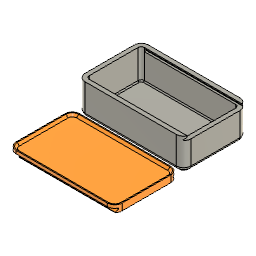
Box+with+Slide+Lid (Autodesk Fusion 360 design; units mm, degrees)
part number: 2025-07-16-15-57-53-406
Autodesk Fusion 360 part; units mm, degrees
note: some values were not read from the file. Set by a fixed rule: which face or edge a step refers to.
sketch "Sketch1" plane through (0, 0, 0) normal (0, 0, 1) x (1, 0, 0)
  line L0 (7, 0) -> (93, 0)
  line L1 (100, 7) -> (100, 53)
  line L2 (93, 60) -> (7, 60)
  line L3 (0, 53) -> (0, 7)
  arc A0 (7, 60) -> (0, 53) centre (7, 53) ccw
  arc A1 (100, 53) -> (93, 60) centre (93, 53) ccw
  arc A2 (93, 0) -> (100, 7) centre (93, 7) ccw
  arc A3 (0, 7) -> (7, 0) centre (7, 7) ccw
  point P0 (100, 0)
  point P1 (0, 60)
  dimension "d5" = 60
  dimension "d6" = 100
  dimension "d7" = 7
  constraint horizontal L0
  constraint vertical L1
  constraint horizontal L2
  constraint vertical L3
  constraint coincident P1 L2
  constraint coincident P1 L3
  constraint tangent L2 A0
  constraint tangent L3 A0
  constraint tangent L1 A1
  constraint tangent L2 A1
  constraint coincident P0 L0
  constraint coincident P0 L1
  constraint tangent L0 A2
  constraint tangent L1 A2
  constraint equal A1 A2
  constraint coincident origin L0
  constraint coincident origin L3
  constraint tangent L0 A3
  constraint tangent L3 A3
  constraint equal A1 A3
  constraint equal A0 A1
  measures "d5" distance of origin P1
  measures "d6" distance of origin P0
  measures "d7" radius of A0
extrude "Extrude1" add sketch "Sketch1" along normal blind 30 makes body 1
shell "Shell1" thickness 4 removed faces 1 at (64.3333, 20, 30) on bodies 1
extrude "Extrude2" cut 1 faces at (64.3333, 21.3333, 4) along direction (0, 0, -1) blind 2 on bodies 1 bodies 1
chamfer "Chamfer1" distance 3 angle 45 8 edges at (2.0503, 2.0503, 0) (50, 0, 0) (97.9497, 2.0503, 0) (100, 30, 0) (97.9497, 57.9497, 0) (50, 60, 0) (2.0503, 57.9497, 0) (0, 30, 0) on bodies 1
fillet "Fillet1" radius 3 8 edges at (2.0503, 57.9497, 3) (50, 60, 3) (97.9497, 57.9497, 3) (100, 30, 3) (97.9497, 2.0503, 3) (50, 0, 3) (2.0503, 2.0503, 3) (0, 30, 3) on bodies 1
chamfer "Chamfer2" distance 1 distance2 1 8 edges at (50, 56, 2) (95.1213, 55.1213, 2) (96, 30, 2) (95.1213, 4.8787, 2) (50, 4, 2) (4.8787, 4.8787, 2) (4, 30, 2) (4.8787, 55.1213, 2) measured on face at (35.6667, 56, 20.6667) measured on face at (94.3747, 55.6665, 11.3333) measured on face at (96, 22.3333, 11.3333) measured on face at (93.2852, 4.0136, 20.6667) measured on face at (35.6667, 4, 11.3333) measured on face at (4.0034, 6.8573, 20.6667) measured on face at (4, 22.3333, 20.6667) measured on face at (5.5, 55.5981, 20.6667) on bodies 1
sketch "Sketch5" plane through (0, 0, 0) normal (0, 0, 1) x (1, 0, 0)
  line L0 (7, -5) -> (93, -5)
  line L1 (100, -12) -> (100, -58)
  line L2 (93, -65) -> (7, -65)
  line L3 (0, -58) -> (0, -12)
  arc A0 (7, -5) -> (0, -12) centre (7, -12) ccw
  arc A1 (100, -12) -> (93, -5) centre (93, -12) ccw
  arc A2 (93, -65) -> (100, -58) centre (93, -58) ccw
  arc A3 (0, -58) -> (7, -65) centre (7, -58) ccw
  point P0 (0, -5)
  point P1 (100, -5)
  point P2 (0, -65)
  dimension "d37" = 100
  dimension "d38" = 60
  dimension "d39" = 5
  dimension "d40" = 7
  constraint horizontal L0
  constraint vertical L1
  constraint horizontal L2
  constraint vertical L3
  constraint coincident P0 L0
  constraint coincident P0 L3
  constraint tangent L0 A0
  constraint tangent L3 A0
  constraint coincident P1 L0
  constraint coincident P1 L1
  constraint tangent L0 A1
  constraint tangent L1 A1
  constraint tangent L1 A2
  constraint tangent L2 A2
  constraint equal A0 A2
  constraint coincident P2 L2
  constraint coincident P2 L3
  constraint tangent L2 A3
  constraint tangent L3 A3
  constraint equal A0 A1
  constraint equal A0 A3
  constraint vertical P0 origin
  measures "d37" distance of P0 P1
  measures "d38" distance of P0 P2
  measures "d39" distance of P0 origin
  measures "d40" radius of A0
extrude "Extrude3" add sketch "Sketch5" along normal blind 1 from surface at 3.5 separate body makes body 2
ref_plane "WorkPlane1" through (50, -35, 4) normal (0, -1, 0) x (1, 0, 0)
sketch "Sketch3" plane through (0, -35, 0) normal (0, -1, 0) x (-1, 0, 0)
  line L0 (0, -4.5) -> (0, -6.5)
  line L1 (0, -6.5) -> (-1, -6.5)
  line L2 (-1, -6.5) -> (-3, -4.5)
  line L3 (-3, -4.5) -> (0, -4.5)
  point P0 (0, -4.5)
  dimension "d42" = 2
  dimension "d43" = 1
  dimension "d44" = 45
  constraint vertical L0
  constraint perpendicular L0 L1
  constraint perpendicular L0 L3
  constraint coincident P0 L0.start
  measures "d42" distance of P0 L0.end
  measures "d43" distance of L0.end L1.end
  measures "d44" angle of L2 L3
sweep "Sweep1" add profiles "Sketch3" along 8 edges at (2.0503, -62.9497, 4.5) (50, -65, 4.5) (97.9497, -62.9497, 4.5) (100, -35, 4.5) (97.9497, -7.0503, 4.5) (50, -5, 4.5) (2.0503, -7.0503, 4.5) (0, -35, 4.5) section 1 on bodies 2 bodies 2
sketch "Sketch6" plane through (100, 0, 0) normal (1, 0, 0) x (0, 1, 0)
  line L0 (-58, 3.5) -> (-12, 3.5)
  line L1 (-12, 3.5) -> (-12, 6.5)
  line L2 (-12, 6.5) -> (-58, 6.5)
  line L3 (-58, 6.5) -> (-58, 3.5)
  line L4 (-35, 3.5) -> (-35, 0)
  line L5 (-35, 0) -> (-62.8, 0)
  line L6 (-62.8, 0) -> (-62.8, 0.4)
  line L7 (-60.8, 3.5) -> (-35, 3.5)
  line L8 (-62.8, 0.4) -> (-60.8, 2.4)
  line L9 (-60.8, 2.4) -> (-60.8, 3.5)
  point P0 (-65, 3.5)
  dimension "d47" = 3.5
  dimension "d48" = 2
  dimension "d50" = 0.4
  dimension "d51" = 1.1
  dimension "d69" = 27.8
  constraint vertical L4
  constraint perpendicular L4 L5
  constraint perpendicular L5 L6
  constraint perpendicular L4 L7
  constraint vertical L9
  constraint midpoint L0 L4.start
  measures "d47" distance of L4.start L4.end
  measures "d48" horizontal distance of L5.end L7.start
  measures "d50" distance of L5.end L6.end
  measures "d51" distance of L7.start L8.end
  measures "d69" distance of L4.end L5.end
extrude "Extrude4" add sketch "Sketch6" against normal blind 92.9 separate body contours L0 L4 L5 L6 L7 L8 L9 makes body 3
mirror "Mirror1" about plane through (100, -35, 3.5) normal (0, 1, 0) of bodies 3 merged
extrude "Extrude5" cut 1 faces at (64.3333, -25, 3.5) along direction (0, 0, -1) blind 4 keep common part on bodies 2 bodies 3
sketch "Sketch8" plane through (0, 0, 3.5) normal (0, 0, -1) x (1, 0, 0)
  arc A0 (0, 12) -> (7, 5) centre (7, 12) ccw
  line L0 (7, 5) -> (93, 5)
  arc A1 (93, 5) -> (100, 12) centre (93, 12) ccw
  line L1 (100, 12) -> (100, 58)
  arc A2 (100, 58) -> (93, 65) centre (93, 58) ccw
  line L2 (93, 65) -> (7, 65)
  arc A3 (7, 65) -> (0, 58) centre (7, 58) ccw
  line L3 (0, 58) -> (0, 12)
  arc A4 (7, 60.8) -> (4.2, 58) centre (7, 58) ccw
  line L4 (4.2, 58) -> (4.2, 12)
  arc A5 (4.2, 12) -> (7, 9.2) centre (7, 12) ccw
  line L5 (7, 60.8) -> (7.1, 60.8)
  line L6 (7.1, 60.8) -> (7.1, 9.2)
  line L7 (7.1, 62.8) -> (7.1, 7.2)
  line L8 (7, 9.2) -> (7.1, 9.2)
  dimension "d66" = -4.2
  constraint tangent A4 L5
  constraint horizontal L5
  constraint perpendicular L5 L6
  constraint coincident L5.end L7
  constraint coincident L7 L6.end
  constraint tangent A5 L8
  constraint horizontal L8
  constraint coincident L6.end L8.end
extrude "Extrude7" add sketch "Sketch8" along normal blind 3.5 contours A4 L4 A5 L5 L6 L7 L8 bodies 2 3
sketch "Sketch7" plane through (100, 0, 0) normal (1, 0, 0) x (0, 1, 0)
  line L0 (7, 4.2426) -> (53, 4.2426)
  line L1 (53, 4.2426) -> (53, 30)
  line L2 (53, 30) -> (7, 30)
  line L3 (7, 30) -> (7, 4.2426)
  line L4 (4, 30) -> (4, 29)
  line L5 (4, 29) -> (2, 27)
  line L6 (2, 27) -> (2, 26.5)
  line L7 (2, 26.5) -> (4, 26.5)
  line L8 (4, 26.5) -> (4, 29)
  line L9 (7, 30) -> (0, 30)
  line L10 (30, 30) -> (30, 26.5) construction
  line L11 (58, 26.5) -> (56, 26.5)
  line L12 (58, 27) -> (58, 26.5)
  line L13 (56, 30) -> (56, 29)
  line L14 (56, 26.5) -> (56, 29)
  line L15 (56, 29) -> (58, 27)
  line L16 (4, 26.5) -> (56, 26.5)
  line L17 (56, 30) -> (4, 30)
  dimension "d59" = 1
  dimension "d60" = 3.5
  dimension "d61" = 4
  dimension "d62" = 0.5
  dimension "d63" = 2
  constraint vertical L4
  constraint parallel L4 L6
  constraint perpendicular L6 L7
  constraint perpendicular L7 L8
  constraint coincident L4.start L9
  constraint coincident L2 L10.start
  constraint perpendicular L7 L10
  constraint horizontal L7.end L10.end
  constraint midpoint L2 L10.start
  constraint symmetric L4.start L10 L13.start
  constraint symmetric L4.end L10 L13.end
  constraint symmetric L5.end L10 L12.start
  constraint symmetric L6.end L10 L11.start
  constraint symmetric L7.end L10 L11.end
  measures "d59" distance of L4.start L4.end
  measures "d60" distance of L4.start L7.end
  measures "d61" distance of L4.start L9.end
  measures "d62" distance of L5.end L6.end
  measures "d63" distance of L6.end L7.end
extrude "Extrude6" cut sketch "Sketch7" against normal blind 93 contours L3 L4 L8 L9 L16 L17 | L1 L2 L3 L16 L17 | L1 L13 L14 L16 L17 | L5 L6 L7 L8 | L11 L12 L14 L15 bodies 1
sketch "Sketch9" plane through (0, 0, 2) normal (0, 0, 1) x (-1, 0, 0)
  line L0 (-93, -55) -> (-7, -55)
  arc A0 (-7, -55) -> (-5, -53) centre (-7, -53) ccw
  line L1 (-5, -53) -> (-5, -7)
  arc A1 (-5, -7) -> (-7, -5) centre (-7, -7) ccw
  line L2 (-7, -5) -> (-93, -5)
  arc A2 (-93, -5) -> (-95, -7) centre (-93, -7) ccw
  line L3 (-95, -7) -> (-95, -53)
  arc A3 (-95, -53) -> (-93, -55) centre (-93, -53) ccw
  line L4 (-3, -56) -> (-3, -4)
  line L5 (-4, -29) -> (-2, -29)
  line L6 (-2, -29) -> (-2, -31)
  line L7 (-2, -31) -> (-4, -31)
  line L8 (-4, -31) -> (-4, -29)
  line L9 (-4, -29) -> (-2, -31) construction
  line L10 (-2, -29) -> (-4, -31) construction
  point P0 (-7, -56)
  point P1 (-7, -4)
  point P2 (-3, -30)
  dimension "d72" = 3
  dimension "d116" = 2
  dimension "d117" = 2
  constraint vertical L4
  constraint horizontal L4.start P0
  constraint horizontal L4.end P1
  constraint horizontal L5
  constraint perpendicular L5 L6
  constraint parallel L5 L7
  constraint parallel L6 L8
  constraint coincident L9 P2
  constraint coincident L10 P2
  constraint midpoint L4 P2
  measures "d72" distance of origin L4
  measures "d116" distance of L6.end L7.end
  measures "d117" distance of L5.end L6.end
extrude "Extrude8" add sketch "Sketch9" along normal blind 24 thin wall 2 centred separate body open curves L4 makes body 4
extrude "Extrude12" add sketch "Sketch9" against normal blind 2 contours L4 L5 L7 L8 | L4 L5 L6 L7 bodies 4
pattern_linear "R-Pattern1" count 1 spacing 94 along (1, 0, 0) of bodies 4 merged
sketch "Sketch10" plane through (0, 0, 2) normal (0, 0, 1) x (-1, 0, 0)
  line L0 (-93, -55) -> (-7, -55)
  arc A0 (-7, -55) -> (-5, -53) centre (-7, -53) ccw
  line L1 (-5, -53) -> (-5, -7)
  arc A1 (-5, -7) -> (-7, -5) centre (-7, -7) ccw
  line L2 (-7, -5) -> (-93, -5)
  arc A2 (-93, -5) -> (-95, -7) centre (-93, -7) ccw
  line L3 (-95, -7) -> (-95, -53)
  arc A3 (-95, -53) -> (-93, -55) centre (-93, -53) ccw
  line L4 (-4, -3) -> (-96, -3)
  line L5 (-51, -2) -> (-49, -2)
  line L6 (-49, -2) -> (-49, -4)
  line L7 (-49, -4) -> (-51, -4)
  line L8 (-51, -4) -> (-51, -2)
  line L9 (-51, -2) -> (-49, -4) construction
  line L10 (-49, -2) -> (-51, -4) construction
  point P0 (-4, -7)
  point P1 (-96, -7)
  point P2 (-50, -3)
  dimension "d82" = 3
  dimension "d120" = 2
  dimension "d121" = 2
  constraint horizontal L4
  constraint vertical L4.start P0
  constraint vertical L4.end P1
  constraint horizontal L5
  constraint perpendicular L5 L6
  constraint parallel L5 L7
  constraint parallel L6 L8
  constraint coincident L9 P2
  constraint coincident L10 P2
  constraint midpoint L4 P2
  measures "d82" distance of origin L4
  measures "d120" distance of L6.end L7.end
  measures "d121" distance of L5.end L6.end
extrude "Extrude9" add sketch "Sketch10" along normal blind 24 thin wall 2 centred separate body open curves L4 makes body 5
extrude "Extrude13" add sketch "Sketch10" against normal blind 2 contours L4 L6 L7 L8 | L4 L5 L6 L8 bodies 5
pattern_linear "R-Pattern2" count 1 spacing 54 along (0, 1, 0) of bodies 5 merged
delete_body "RemoveBody1" bodies 4
delete_body "RemoveBody2" bodies 5
sketch "Sketch11" plane through (0, 0, 0) normal (0, 0, -1) x (1, 0, 0)
  arc A0 (100, 58) -> (98.0951, 62.8) centre (93, 58) ccw
  line L0 (98.0951, 62.8) -> (7.1, 62.8)
  line L1 (7.1, 62.8) -> (7.1, 60.8)
  arc A1 (7, 60.8) -> (4.2, 58) centre (7, 58) ccw
  line L2 (4.2, 58) -> (4.2, 12)
  line L3 (7.1, 7.2) -> (98.0951, 7.2)
  arc A2 (98.0951, 7.2) -> (100, 12) centre (93, 12) ccw
  line L4 (100, 12) -> (100, 58)
  line L5 (8.75, 7.2) -> (9.2647, 7.4745)
  line L6 (9.7353, 7.4745) -> (10.25, 7.2)
  line L7 (8.75, 7.2) -> (10.25, 7.2)
  arc A3 (7.1, 7.7) -> (7.6, 7.2) centre (7.6, 7.7) ccw
  line L8 (7.1, 7.7) -> (7.1, 7.2)
  line L9 (7.6, 7.2) -> (7.1, 7.2)
  arc A4 (9.7353, 7.4745) -> (9.2647, 7.4745) centre (9.5, 7.0333) ccw
  line L10 (4.2, 35) -> (14.2, 35) construction
  arc A5 (9.2647, 62.5255) -> (9.7353, 62.5255) centre (9.5, 62.9667) ccw
  arc A6 (7.6, 62.8) -> (7.1, 62.3) centre (7.6, 62.3) ccw
  line L11 (9.7353, 62.5255) -> (10.25, 62.8)
  line L12 (7.6, 62.8) -> (7.1, 62.8)
  line L13 (8.75, 62.8) -> (10.25, 62.8)
  line L14 (7.1, 62.3) -> (7.1, 62.8)
  line L15 (8.75, 62.8) -> (9.2647, 62.5255)
  line L16 (7, 8) -> (7, 6)
  point P0 (9.5, 7.6)
  point P1 (9.5, 62.4)
  point P2 (25.1, 50.8)
  dimension "d94" = 0.4
  dimension "d97" = 0.5
  dimension "d98" = 0.5
  dimension "d100" = 10
  dimension "d112" = 1.5
  dimension "d114" = 2.5
  constraint coincident L3 L5.start
  constraint coincident L3 L6.end
  constraint coincident L3.start L8.end
  constraint tangent A3 L8
  constraint tangent A3 L9
  constraint coincident L3 A3.end
  constraint vertical L8
  constraint coincident P0 L5
  constraint coincident P0 L6
  constraint tangent L5 A4
  constraint tangent L6 A4
  constraint midpoint L2 L10.start
  constraint perpendicular L2 L10
  constraint symmetric L5.start L10 L13.start
  constraint symmetric P0 L10 P1
  constraint symmetric L6.end L10 L11.end
  constraint symmetric A3.start L10 A6.end
  constraint symmetric A3.end L10 A6.start
  constraint symmetric A3 L10 A6
  constraint symmetric L3.start L10 L0.end
  constraint symmetric L5.end L10 A5.start
  constraint symmetric L6.start L10 A5.end
  constraint symmetric A4 L10 A5
  constraint equal L5 L6
  measures "d94" distance of P0 L7
  measures "d97" radius of A3
  measures "d98" radius of A4
  measures "d100" distance of L10.start L10.end
  measures "d112" distance of L5.start L6.end
  measures "d114" distance of A4.centre L16
extrude "Extrude10" cut sketch "Sketch11" against normal blind 3 bodies 2
sketch "Sketch12" plane through (0, 0, 30) normal (0, 0, 1) x (-1, 0, 0)
  line L0 (-99.3246, -4) -> (-7, -4)
  arc A0 (-4, -7) -> (-7, -4) centre (-7, -7) ccw
  line L1 (-4, -7) -> (-4, -53)
  arc A1 (-7, -56) -> (-4, -53) centre (-7, -53) ccw
  line L2 (-7, -56) -> (-99.3246, -56)
  arc A2 (-99.3246, -56) -> (-93, -60) centre (-93, -53) ccw
  line L3 (-93, -60) -> (-7, -60)
  arc A3 (-7, -60) -> (0, -53) centre (-7, -53) ccw
  line L4 (0, -53) -> (0, -7)
  arc A4 (0, -7) -> (-7, 0) centre (-7, -7) ccw
  line L5 (-7, 0) -> (-93, 0)
  arc A5 (-93, 0) -> (-99.3246, -4) centre (-93, -7) ccw
  line L6 (-8.75, -2) -> (-9.2647, -2.2745)
  line L7 (-9.7353, -2.2745) -> (-10.25, -2)
  line L8 (-10.25, -2) -> (-8.75, -2)
  line L9 (-7, -4) -> (-7, -5)
  line L10 (-97.899, -2) -> (-7, -2)
  arc A6 (-9.7353, -2.2745) -> (-9.2647, -2.2745) centre (-9.5, -1.8333) ccw
  line L11 (-4, -30) -> (-14, -30) construction
  line L12 (-10.25, -58) -> (-8.75, -58)
  line L13 (-9.7353, -57.7255) -> (-10.25, -58)
  arc A7 (-9.2647, -57.7255) -> (-9.7353, -57.7255) centre (-9.5, -58.1667) ccw
  line L14 (-8.75, -58) -> (-9.2647, -57.7255)
  point P0 (-9.5, -2.4)
  point P1 (-14, -30)
  point P2 (-9.5, -57.6)
  dimension "d105" = 0.4
  dimension "d106" = 2.5
  dimension "d107" = 0.5
  dimension "d108" = 10
  dimension "d115" = 1.5
  constraint parallel L0 L8
  constraint coincident L6.start L10
  constraint coincident P0 L6
  constraint coincident P0 L7
  constraint tangent L6 A6
  constraint tangent L7 A6
  constraint midpoint L1 L11.start
  constraint perpendicular L1 L11
  constraint symmetric L6.start L11 L12.end
  constraint symmetric P0 L11 P2
  constraint symmetric L7.end L11 L12.start
  constraint symmetric L6.end L11 A7.start
  constraint symmetric L7.start L11 L13.start
  constraint symmetric A6 L11 A7
  constraint symmetric P1 L11 L11.end
  constraint equal L6 L7
  measures "d105" distance of P0 L8
  measures "d106" distance of P0 L9
  measures "d107" radius of A6
  measures "d108" distance of L11.start P1
  measures "d115" distance of L6.start L7.end
extrude "Extrude11" add sketch "Sketch12" against normal blind 4 contours L6 L7 L8 L10 A6 | L12 L13 A7 L14 bodies 1
equation "Length = 100 mm"
equation "Width = 60 mm"
equation "CornerRadius = 7 mm"
equation "Height = 30 mm"
equation "d5 = Width"
equation "d6 = Length"
equation "d7 = CornerRadius"
equation "Thickness = 4 mm"
equation "d10 = Height"
equation "d12 = Thickness"
equation "d13 = -Thickness + 2 mm"
equation "d37 = Length"
equation "d38 = Width"
equation "d40 = CornerRadius"
equation "d52 = -Length + CornerRadius + 0.1 mm"
equation "d64 = -Length + CornerRadius"
equation "d69 = ( Width / 2 ) - 2.2 mm"
equation "LengthSection = 1"
equation "WidthSection = 1"
equation "d74 = Height - 6 mm"
equation "LengthSectionDistance = ( Length - 6 mm ) / LengthSection"
equation "WidthSectionDistance = ( Width - 6 mm ) / WidthSection"
equation "d78 = LengthSection"
equation "d80 = -LengthSectionDistance"
equation "d84 = Height - 6 mm"
equation "d86 = WidthSection"
equation "d88 = -WidthSectionDistance"
named bodies: "Box", "Lid"
